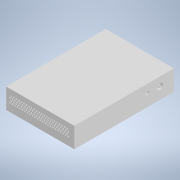
# Autodesk Inventor part: UBIQUITI EDGEROUTER-X
Saved by Autodesk Inventor 2020.2 (Build 242310000, 310)
## iProperties
Created: 2020-02-16
Part Number: UBIQUITI EDGEROUTER-X
Material: Generic
Document SubType Name: Modeling
Designer: mulve
Density: 1 g/cm^3
Appearance: Default
Author: mulve
Autodesk Inventor part; units mm, degrees
ref_plane "YZ Plane" through (0, 0, 0) normal (1, 0, 0) x (0, 1, 0)
ref_plane "XZ Plane" through (0, 0, 0) normal (0, 1, 0) x (-1, 0, 0)
sketch "Sketch1" plane through (0, 0, 0) normal (0, 1, 0) x (-1, 0, 0)
  line L0 (0, 0) -> (75.65, 0)
  line L1 (75.65, 0) -> (75.65, -110.31)
  line L2 (75.65, -110.31) -> (0, -110.31)
  line L3 (0, -110.31) -> (0, 0)
  dimension "d0" = 110.31
  dimension "d1" = 75.65
  constraints: 8 end point, 2 parallel, 1 horizontal, 1 perpendicular
  measures "d0" distance of L2.end L0.start
  measures "d1" distance of L1.end L2.end
extrude "Extrusion1" add sketch "Sketch1" along normal blind 22.5
sketch "Sketch2" plane through (0, 0, 0) normal (1, 0, 0) x (0, 0, -1)
  line L0 (0, 22.5) -> (110.31, 22.5) projected
  line L1 (0, 0) -> (0, 22.5) projected
  line L2 (110.31, 0) -> (110.31, 22.5) projected
  circle A0 centre (5.54, 15.27) radius 1.925
  circle A1 centre (104.77, 15.27) radius 1.925
  dimension "d4" = 7.23
  dimension "d5" = 7.23
  dimension "d6" = 5.54
  dimension "d7" = 5.54
  dimension "d8" = 3.85
  constraints: 2 centre point, 2 coincident, 1 equal radius
  measures "d4" distance from line of L0 point (5.54, 15.27)
  measures "d5" distance from line of L0 point (104.77, 15.27)
  measures "d6" distance from line of L1 point (5.54, 15.27)
  measures "d7" distance from line of L2 point (104.77, 15.27)
  measures "d8" diameter of A0
extrude "Extrusion2" cut sketch "Sketch2" against normal blind 0.1
sketch "Sketch3" plane through (0, 0, 0) normal (1, 0, 0) x (0, 0, -1)
  line L0 (0, 22.5) -> (110.31, 22.5) projected
  line L1 (0, 0) -> (0, 22.5) projected
  circle A0 centre (81.06, 13.3) radius 1.875
  dimension "d11" = 9.2
  dimension "d12" = 81.06
  dimension "d13" = 3.75
  constraints: 1 centre point, 1 coincident
  measures "d11" distance from line of L0 point (81.06, 13.3)
  measures "d12" distance from line of L1 point (81.06, 13.3)
  measures "d13" diameter of A0
extrude "Extrusion3" cut sketch "Sketch3" against normal blind 12.7
sketch "Sketch4" plane through (0, 0, 0) normal (1, 0, 0) x (0, 0, -1)
  line L0 (0, 0) -> (0, 22.5) projected
  line L1 (0, 22.5) -> (110.31, 22.5) projected
  circle A0 centre (13.8, 9.13) radius 1.5
  dimension "d16" = 13.8
  dimension "d17" = 13.37
  dimension "d18" = 3
  constraints: 1 centre point, 1 coincident
  measures "d16" distance from line of L0 point (13.8, 9.13)
  measures "d17" distance from line of L1 point (13.8, 9.13)
  measures "d18" diameter of A0
extrude "Extrusion4" cut sketch "Sketch4" against normal blind 0.2
sketch "Sketch5" plane through (0, 0, 0) normal (1, 0, 0) x (0, 0, -1)
  line L0 (90.8, 16.86) -> (99.47, 16.86)
  line L1 (99.47, 16.86) -> (99.47, 5.38)
  line L2 (99.47, 5.38) -> (90.8, 5.38)
  line L3 (90.8, 5.38) -> (90.8, 16.86)
  line L4 (110.31, 0) -> (110.31, 22.5) projected
  line L5 (0, 22.5) -> (110.31, 22.5) projected
  circle A0 centre (95.135, 12.62) radius 3.24
  circle A1 centre (95.135, 12.62) radius 1.125
  point P0 (0, 0)
  point P1 (95.135, 15.86)
  dimension "d25" = 6.48
  dimension "d21" = 8.67
  dimension "d22" = 10.84
  dimension "d23" = 11.48
  dimension "d24" = 5.64
  dimension "d26" = 1
  dimension "d27" = 2.25
  constraints: 8 end point, 2 coincident, 2 parallel, 1 centre point, 1 horizontal, 1 perpendicular, 1 vertical alignment, 2 other
  measures "d21" distance of L1.end L2.end
  measures "d22" distance between parallel lines of L4 L1
  measures "d23" distance of L0.end L1.end
  measures "d24" distance between parallel lines of L5 L0
  measures "d26" distance from line of L0 point (95.135, 15.86)
  measures "d27" diameter of A1
extrude "Extrusion5" cut sketch "Sketch5" against normal blind 9.2 contours A0
sketch "Sketch7" plane through (-75.65, 0, -110.31) normal (-1, 0, 0) x (0, 0, 1)
  line L0 (8.57, 5.39) -> (25.73, 5.39)
  line L1 (25.73, 5.39) -> (25.73, 19.5)
  line L2 (25.73, 19.5) -> (8.57, 19.5)
  line L3 (8.57, 19.5) -> (8.57, 5.39)
  line L4 (0, 22.5) -> (110.31, 22.5) projected
  line L5 (0, 0) -> (0, 22.5) projected
  line L6 (44.78, 5.39) -> (44.78, 19.5)
  line L7 (44.78, 19.5) -> (27.62, 19.5)
  line L8 (27.62, 19.5) -> (27.62, 5.39)
  line L9 (27.62, 5.39) -> (44.78, 5.39)
  line L10 (63.83, 5.39) -> (63.83, 19.5)
  line L11 (63.83, 19.5) -> (46.67, 19.5)
  line L12 (46.67, 19.5) -> (46.67, 5.39)
  line L13 (46.67, 5.39) -> (63.83, 5.39)
  line L14 (82.88, 5.39) -> (82.88, 19.5)
  line L15 (82.88, 19.5) -> (65.72, 19.5)
  line L16 (65.72, 19.5) -> (65.72, 5.39)
  line L17 (65.72, 5.39) -> (82.88, 5.39)
  line L18 (101.93, 5.39) -> (101.93, 19.5)
  line L19 (101.93, 19.5) -> (84.77, 19.5)
  line L20 (84.77, 19.5) -> (84.77, 5.39)
  line L21 (84.77, 5.39) -> (101.93, 5.39)
  point P0 (110.31, 0)
  dimension "d30" = 17.16
  dimension "d31" = 14.11
  dimension "d32" = 3
  dimension "d33" = 8.57
  dimension "d36" = 19.05
  constraints: 40 end point, 2 horizontal, 2 parallel, 1 perpendicular, 32 other
  measures "d30" distance of L1.end L2.end
  measures "d31" distance of L0.end L1.end
  measures "d32" distance between parallel lines of L4 L2
  measures "d33" distance between parallel lines of L5 L3
  measures "d36" distance of L0.end L6.start
extrude "Extrusion6" cut sketch "Sketch7" against normal blind 0.1
sketch "Sketch8" plane through (-75.55, 0, -110.31) normal (-1, 0, 0) x (0, 0, 1)
  line L0 (11.1, 7.46) -> (23.2, 7.46)
  line L1 (23.2, 7.46) -> (23.2, 14.99)
  line L2 (23.2, 14.99) -> (11.1, 14.99)
  line L3 (11.1, 14.99) -> (11.1, 7.46)
  line L4 (8.57, 5.39) -> (8.57, 19.5) projected
  line L5 (25.73, 19.5) -> (25.73, 5.39) projected
  line L6 (25.73, 5.39) -> (8.57, 5.39) projected
  line L7 (13.815, 7.46) -> (20.485, 7.46)
  line L8 (20.485, 7.46) -> (20.485, 16.67)
  line L9 (20.485, 16.67) -> (13.815, 16.67)
  line L10 (13.815, 16.67) -> (13.815, 7.46)
  line L11 (15.055, 7.46) -> (19.245, 7.46)
  line L12 (19.245, 7.46) -> (19.245, 18.23)
  line L13 (19.245, 18.23) -> (15.055, 18.23)
  line L14 (15.055, 18.23) -> (15.055, 7.46)
  line L15 (34.155, 18.23) -> (34.155, 7.46)
  line L16 (30.2, 14.99) -> (30.2, 7.46)
  line L17 (32.915, 16.67) -> (32.915, 7.46)
  line L18 (38.345, 7.46) -> (38.345, 18.23)
  line L19 (39.585, 7.46) -> (39.585, 16.67)
  line L20 (42.3, 7.46) -> (42.3, 14.99)
  line L21 (38.345, 18.23) -> (34.155, 18.23)
  line L22 (39.585, 16.67) -> (32.915, 16.67)
  line L23 (42.3, 14.99) -> (30.2, 14.99)
  line L24 (34.155, 7.46) -> (38.345, 7.46)
  line L25 (30.2, 7.46) -> (42.3, 7.46)
  line L26 (53.255, 18.23) -> (53.255, 7.46)
  line L27 (49.3, 14.99) -> (49.3, 7.46)
  line L28 (52.015, 16.67) -> (52.015, 7.46)
  line L29 (57.445, 7.46) -> (57.445, 18.23)
  line L30 (58.685, 7.46) -> (58.685, 16.67)
  line L31 (61.4, 7.46) -> (61.4, 14.99)
  line L32 (57.445, 18.23) -> (53.255, 18.23)
  line L33 (58.685, 16.67) -> (52.015, 16.67)
  line L34 (61.4, 14.99) -> (49.3, 14.99)
  line L35 (53.255, 7.46) -> (57.445, 7.46)
  line L36 (49.3, 7.46) -> (61.4, 7.46)
  line L37 (72.355, 18.23) -> (72.355, 7.46)
  line L38 (68.4, 14.99) -> (68.4, 7.46)
  line L39 (71.115, 16.67) -> (71.115, 7.46)
  line L40 (76.545, 7.46) -> (76.545, 18.23)
  line L41 (77.785, 7.46) -> (77.785, 16.67)
  line L42 (80.5, 7.46) -> (80.5, 14.99)
  line L43 (76.545, 18.23) -> (72.355, 18.23)
  line L44 (77.785, 16.67) -> (71.115, 16.67)
  line L45 (80.5, 14.99) -> (68.4, 14.99)
  line L46 (72.355, 7.46) -> (76.545, 7.46)
  line L47 (68.4, 7.46) -> (80.5, 7.46)
  line L48 (91.455, 18.23) -> (91.455, 7.46)
  line L49 (87.5, 14.99) -> (87.5, 7.46)
  line L50 (90.215, 16.67) -> (90.215, 7.46)
  line L51 (95.645, 7.46) -> (95.645, 18.23)
  line L52 (96.885, 7.46) -> (96.885, 16.67)
  line L53 (99.6, 7.46) -> (99.6, 14.99)
  line L54 (95.645, 18.23) -> (91.455, 18.23)
  line L55 (96.885, 16.67) -> (90.215, 16.67)
  line L56 (99.6, 14.99) -> (87.5, 14.99)
  line L57 (91.455, 7.46) -> (95.645, 7.46)
  line L58 (87.5, 7.46) -> (99.6, 7.46)
  point P0 (110.31, 0)
  point P1 (91.455, 16.67)
  point P2 (90.215, 14.99)
  point P3 (91.455, 7.46)
  point P4 (96.885, 14.99)
  point P5 (95.645, 16.67)
  point P6 (77.785, 14.99)
  point P7 (76.545, 16.67)
  point P8 (72.355, 16.67)
  point P9 (71.115, 14.99)
  point P10 (72.355, 7.46)
  point P11 (53.255, 7.46)
  point P12 (58.685, 14.99)
  point P13 (57.445, 16.67)
  point P14 (53.255, 16.67)
  point P15 (52.015, 14.99)
  point P16 (39.585, 14.99)
  point P17 (38.345, 16.67)
  point P18 (34.155, 16.67)
  point P19 (32.915, 14.99)
  point P20 (34.155, 7.46)
  point P21 (15.055, 16.67)
  point P22 (13.815, 14.99)
  point P23 (20.485, 14.99)
  point P24 (19.245, 16.67)
  dimension "d43" = 12.1
  dimension "d45" = 2.53
  dimension "d46" = 2.53
  dimension "d47" = 2.07
  dimension "d48" = 6.67
  dimension "d50" = 2.715
  dimension "d51" = 2.715
  dimension "d52" = 4.19
  dimension "d53" = 12.84
  dimension "d54" = 11.28
  dimension "d55" = 9.6
  dimension "d56" = 1.24
  dimension "d57" = 1.24
  dimension "d60" = 19.1
  constraints: 112 end point, 6 parallel, 6 point on line, 4 horizontal, 3 perpendicular, 1 collinear, 91 other
  measures "d43" distance of L0.start L0.end
  measures "d45" distance between parallel lines of L4 L3
  measures "d46" distance between parallel lines of L5 L1
  measures "d47" distance between parallel lines of L6 L0
  measures "d48" distance of L8.end L9.end
  measures "d50" distance between parallel lines of L3 L10
  measures "d51" distance between parallel lines of L1 L8
  measures "d52" distance of L12.end L13.end
  measures "d53" distance between parallel lines of L6 L13
  measures "d54" distance between parallel lines of L6 L9
  measures "d55" distance between parallel lines of L6 L2
  measures "d56" distance between parallel lines of L10 L14
  measures "d57" distance between parallel lines of L8 L12
  measures "d60" distance of L13.end L15.start
extrude "Extrusion7" cut sketch "Sketch8" against normal blind 15.75
sketch "Sketch9" plane through (0, 22.5, 0) normal (0, 1, 0) x (1, 0, 0)
  line L0 (0, 0) -> (0, 110.31) projected
  line L1 (0, 110.31) -> (-75.65, 110.31) projected
  circle A0 centre (-5.6, 88.05) radius 0.83
  circle A1 centre (-5.6, 74.79) radius 0.83
  circle A2 centre (-5.6, 65.06) radius 0.83
  circle A3 centre (-5.6, 55) radius 0.83
  circle A4 centre (-5.6, 45.05) radius 0.83
  circle A5 centre (-5.6, 34.75) radius 0.83
  dimension "d67" = 5.6
  dimension "d68" = 5.6
  dimension "d69" = 5.6
  dimension "d70" = 5.6
  dimension "d71" = 5.6
  dimension "d72" = 22.26
  dimension "d73" = 35.52
  dimension "d74" = 45.25
  dimension "d75" = 55.31
  dimension "d76" = 65.26
  dimension "d77" = 5.6
  dimension "d78" = 75.56
  dimension "d79" = 1.66
  constraints: 6 centre point, 6 coincident, 5 equal radius
  measures "d67" distance from line of L0 point (-5.6, 88.05)
  measures "d68" distance from line of L0 point (-5.6, 74.79)
  measures "d69" distance from line of L0 point (-5.6, 65.06)
  measures "d70" distance from line of L0 point (-5.6, 55)
  measures "d71" distance from line of L0 point (-5.6, 45.05)
  measures "d72" distance from line of L1 point (-5.6, 88.05)
  measures "d73" distance from line of L1 point (-5.6, 74.79)
  measures "d74" distance from line of L1 point (-5.6, 65.06)
  measures "d75" distance from line of L1 point (-5.6, 55)
  measures "d76" distance from line of L1 point (-5.6, 45.05)
  measures "d77" distance from line of L0 point (-5.6, 34.75)
  measures "d78" distance from line of L1 point (-5.6, 34.75)
  measures "d79" diameter of A0
extrude "Extrusion8" cut sketch "Sketch9" against normal blind 0.1
sketch "Sketch10" plane through (0, 0, 0) normal (0, -1, 0) x (1, 0, 0)
  line L0 (0, 0) -> (0, -110.31) projected
  line L1 (-75.65, 0) -> (0, 0) projected
  circle A0 centre (-9.5, -13.8) radius 4.3
  circle A1 centre (-9.5, -95.08) radius 4.3
  circle A2 centre (-55.22, -13.8) radius 4.3
  circle A3 centre (-55.22, -95.08) radius 4.3
  dimension "d82" = 9.5
  dimension "d83" = 13.8
  dimension "d84" = 8.6
  dimension "d87" = 81.28
  dimension "d90" = 45.72
  constraints: 4 centre point, 1 coincident, 1 horizontal, 1 vertical, 6 other
  measures "d82" distance from line of L0 point (-9.5, -13.8)
  measures "d83" distance from line of L1 point (-9.5, -13.8)
  measures "d84" diameter of A0
  measures "d87" distance of A0.centre A1.centre
  measures "d90" distance of A0.centre A2.centre
extrude "Extrusion9" cut sketch "Sketch10" against normal blind 0.33
sketch "Sketch11" plane through (-9.5, 0.33, -13.8) normal (0, -1, 0) x (1, 0, 0)
  circle A0 centre (0, 0) radius 3.825
  line L0 (9.5, 13.8) -> (9.5, -96.51) projected
  line L1 (9.5, -26.4546) -> (9.5, -62.5532)
  line L2 (-14.9441, 13.8) -> (-34.0604, 13.8)
  circle A1 centre (0, -81.3) radius 3.825
  circle A2 centre (-45.7, 0) radius 3.825
  circle A3 centre (-45.7, -81.3) radius 3.825
  dimension "d95" = 7.65
  dimension "d98" = 81.3
  dimension "d101" = 45.7
  constraints: 4 centre point, 4 end point, 2 horizontal, 2 point on line, 1 vertical, 6 other
  measures "d95" diameter of A0
  measures "d98" distance of A0.centre A1.centre
  measures "d101" distance of A0.centre A2.centre
extrude "Extrusion10" add sketch "Sketch11" along normal blind 1.91
fillet "Fillet1" radius 3.82 4 edges at (-13.325, -1.58, -13.8) (-59.025, -1.58, -13.8) (-13.325, -1.58, -95.1) (-59.025, -1.58, -95.1)
sketch "Sketch12" plane through (0, 0, 0) normal (0, -1, 0) x (1, 0, 0)
  line L0 (-34.3649, -13.3738) -> (-34.3649, -29.4338) construction
  line L1 (-32.3449, -15.3938) -> (-32.3449, -27.4138)
  line L2 (-36.3849, -27.4138) -> (-36.3849, -15.3938)
  arc A0 (-32.3449, -15.3938) -> (-36.3849, -15.3938) centre (-34.3649, -15.3938) ccw
  arc A1 (-36.3849, -27.4138) -> (-32.3449, -27.4138) centre (-34.3649, -27.4138) ccw
  line L3 (-42.3899, -21.4038) -> (-26.3399, -21.4038) construction
  line L4 (-40.3699, -23.4238) -> (-28.3599, -23.4238)
  line L5 (-28.3599, -19.3838) -> (-40.3699, -19.3838)
  arc A2 (-40.3699, -19.3838) -> (-40.3699, -23.4238) centre (-40.3699, -21.4038) ccw
  arc A3 (-28.3599, -23.4238) -> (-28.3599, -19.3838) centre (-28.3599, -21.4038) ccw
  circle A4 centre (-34.3649, -21.4038) radius 4
  line L6 (0, 0) -> (0, -110.31) construction
  line L7 (0, -55.155) -> (-75.6763, -55.155) construction
  line L8 (-75.55, -57.055) -> (-75.55, -52.865) construction
  line L9 (-34.3649, -96.9362) -> (-34.3649, -80.8762) construction
  line L10 (-32.3449, -94.9162) -> (-32.3449, -82.8962)
  line L11 (-36.3849, -82.8962) -> (-36.3849, -94.9162)
  arc A5 (-36.3849, -94.9162) -> (-32.3449, -94.9162) centre (-34.3649, -94.9162) ccw
  arc A6 (-32.3449, -82.8962) -> (-36.3849, -82.8962) centre (-34.3649, -82.8962) ccw
  line L12 (-42.3899, -88.9062) -> (-26.3399, -88.9062) construction
  line L13 (-40.3699, -86.8862) -> (-28.3599, -86.8862)
  line L14 (-28.3599, -90.9262) -> (-40.3699, -90.9262)
  arc A7 (-40.3699, -86.8862) -> (-40.3699, -90.9262) centre (-40.3699, -88.9062) ccw
  arc A8 (-28.3599, -90.9262) -> (-28.3599, -86.8862) centre (-28.3599, -88.9062) ccw
  circle A9 centre (-34.3649, -88.9062) radius 4
  point P0 (-29.4304, -19.3838)
  point P1 (-36.3849, -26.4943)
  point P2 (-29.4304, -90.9262)
  point P3 (-36.3849, -83.8157)
  point P4 (-36.3849, -85.4537)
  point P5 (-37.8174, -86.8862)
  point P6 (-37.8174, -90.9262)
  point P7 (-36.3849, -92.3586)
  point P8 (-32.3449, -92.3586)
  point P9 (-30.9124, -90.9262)
  point P10 (-30.9124, -86.8862)
  point P11 (-32.3449, -85.4537)
  point P12 (-30.9124, -19.3838)
  point P13 (-32.3449, -17.9514)
  point P14 (-36.3849, -17.9514)
  point P15 (-37.8174, -19.3838)
  point P16 (-37.8174, -23.4238)
  point P17 (-36.3849, -24.8563)
  point P18 (-32.3449, -24.8563)
  point P19 (-30.9124, -23.4238)
  dimension "d107" = 16.06
  dimension "d108" = 2.02
  dimension "d109" = 16.05
  dimension "d110" = 2.02
  dimension "d111" = 8.03
  dimension "d112" = 8
  dimension "d113" = 8.025
  constraints: 34 end point, 24 point on circle, 21 symmetric about line, 10 centre point, 8 point on line, 8 tangent, 3 midpoint, 2 coincident, 2 parallel, 2 perpendicular, 1 vertical, 5 other
  measures "d107" distance of L0.end L0.start
  measures "d108" horizontal distance of L0.end point (-36.385, -26.494)
  measures "d109" distance of L3.start L3.end
  measures "d110" vertical distance of L3.end point (-29.43, -19.384)
  measures "d111" vertical distance of L0.start L3.end
  measures "d112" diameter of A4
  measures "d113" horizontal distance of L0.start L3.end
extrude "Extrusion11" cut sketch "Sketch12" against normal blind 3.08
sketch "Sketch13" plane through (0, 3.08, 0) normal (0, -1, 0) x (1, 0, 0)
  line L0 (-23.1034, -9.3195) -> (-45.2023, -9.3195)
  line L1 (-45.2023, -9.3195) -> (-45.2023, -32.5345)
  line L2 (-45.2023, -32.5345) -> (-23.1034, -32.5345)
  line L3 (-23.1034, -32.5345) -> (-23.1034, -9.3195)
  line L4 (-23.1034, -102.1795) -> (-45.2023, -102.1795)
  line L5 (-45.2023, -102.1795) -> (-45.2023, -76.0626)
  line L6 (-45.2023, -76.0626) -> (-23.1034, -76.0626)
  line L7 (-23.1034, -76.0626) -> (-23.1034, -102.1795)
  point P0 (0, 0)
  constraints: 16 end point, 4 parallel, 2 horizontal, 2 perpendicular, 2 point on line
extrude "Extrusion12" cut sketch "Sketch13" along normal blind 2
sketch "Sketch14" plane through (-75.65, 0, 0) normal (0, 0, 1) x (1, 0, 0)
  line L0 (0, 22.5) -> (75.65, 22.5) projected
  line L1 (75.65, 0) -> (75.65, 22.5) projected
  circle A0 centre (67.58, 16.07) radius 0.8202
  circle A1 centre (64.76, 16.07) radius 0.8202
  circle A2 centre (61.94, 16.07) radius 0.8202
  circle A3 centre (59.12, 16.07) radius 0.8202
  circle A4 centre (56.3, 16.07) radius 0.8202
  circle A5 centre (53.48, 16.07) radius 0.8202
  circle A6 centre (50.66, 16.07) radius 0.8202
  circle A7 centre (47.84, 16.07) radius 0.8202
  circle A8 centre (45.02, 16.07) radius 0.8202
  circle A9 centre (42.2, 16.07) radius 0.8202
  circle A10 centre (39.38, 16.07) radius 0.8202
  circle A11 centre (36.56, 16.07) radius 0.8202
  circle A12 centre (33.74, 16.07) radius 0.8202
  circle A13 centre (30.92, 16.07) radius 0.8202
  circle A14 centre (28.1, 16.07) radius 0.8202
  circle A15 centre (25.28, 16.07) radius 0.8202
  circle A16 centre (22.46, 16.07) radius 0.8202
  circle A17 centre (19.64, 16.07) radius 0.8202
  circle A18 centre (16.82, 16.07) radius 0.8202
  circle A19 centre (14, 16.07) radius 0.8202
  circle A20 centre (11.18, 16.07) radius 0.8202
  circle A21 centre (8.36, 16.07) radius 0.8202
  circle A22 centre (5.54, 16.07) radius 0.8202
  circle A23 centre (67.58, 11.365) radius 0.8202
  circle A24 centre (64.76, 11.365) radius 0.8202
  circle A25 centre (61.94, 11.365) radius 0.8202
  circle A26 centre (59.12, 11.365) radius 0.8202
  circle A27 centre (56.3, 11.365) radius 0.8202
  circle A28 centre (53.48, 11.365) radius 0.8202
  circle A29 centre (50.66, 11.365) radius 0.8202
  circle A30 centre (47.84, 11.365) radius 0.8202
  circle A31 centre (45.02, 11.365) radius 0.8202
  circle A32 centre (42.2, 11.365) radius 0.8202
  circle A33 centre (39.38, 11.365) radius 0.8202
  circle A34 centre (36.56, 11.365) radius 0.8202
  circle A35 centre (33.74, 11.365) radius 0.8202
  circle A36 centre (30.92, 11.365) radius 0.8202
  circle A37 centre (28.1, 11.365) radius 0.8202
  circle A38 centre (25.28, 11.365) radius 0.8202
  circle A39 centre (22.46, 11.365) radius 0.8202
  circle A40 centre (19.64, 11.365) radius 0.8202
  circle A41 centre (16.82, 11.365) radius 0.8202
  circle A42 centre (14, 11.365) radius 0.8202
  circle A43 centre (11.18, 11.365) radius 0.8202
  circle A44 centre (8.36, 11.365) radius 0.8202
  circle A45 centre (5.54, 11.365) radius 0.8202
  circle A46 centre (68.85, 13.77) radius 0.8202
  circle A47 centre (66.03, 13.77) radius 0.8202
  circle A48 centre (63.21, 13.77) radius 0.8202
  circle A49 centre (60.39, 13.77) radius 0.8202
  circle A50 centre (57.57, 13.77) radius 0.8202
  circle A51 centre (54.75, 13.77) radius 0.8202
  circle A52 centre (51.93, 13.77) radius 0.8202
  circle A53 centre (49.11, 13.77) radius 0.8202
  circle A54 centre (46.29, 13.77) radius 0.8202
  circle A55 centre (43.47, 13.77) radius 0.8202
  circle A56 centre (40.65, 13.77) radius 0.8202
  circle A57 centre (37.83, 13.77) radius 0.8202
  circle A58 centre (35.01, 13.77) radius 0.8202
  circle A59 centre (32.19, 13.77) radius 0.8202
  circle A60 centre (29.37, 13.77) radius 0.8202
  circle A61 centre (26.55, 13.77) radius 0.8202
  circle A62 centre (23.73, 13.77) radius 0.8202
  circle A63 centre (20.91, 13.77) radius 0.8202
  circle A64 centre (18.09, 13.77) radius 0.8202
  circle A65 centre (15.27, 13.77) radius 0.8202
  circle A66 centre (12.45, 13.77) radius 0.8202
  circle A67 centre (9.63, 13.77) radius 0.8202
  circle A68 centre (6.81, 13.77) radius 0.8202
  circle A69 centre (3.99, 13.77) radius 0.8202
  circle A70 centre (68.85, 9.065) radius 0.8202
  circle A71 centre (66.03, 9.065) radius 0.8202
  circle A72 centre (63.21, 9.065) radius 0.8202
  circle A73 centre (60.39, 9.065) radius 0.8202
  circle A74 centre (57.57, 9.065) radius 0.8202
  circle A75 centre (54.75, 9.065) radius 0.8202
  circle A76 centre (51.93, 9.065) radius 0.8202
  circle A77 centre (49.11, 9.065) radius 0.8202
  circle A78 centre (46.29, 9.065) radius 0.8202
  circle A79 centre (43.47, 9.065) radius 0.8202
  circle A80 centre (40.65, 9.065) radius 0.8202
  circle A81 centre (37.83, 9.065) radius 0.8202
  circle A82 centre (35.01, 9.065) radius 0.8202
  circle A83 centre (32.19, 9.065) radius 0.8202
  circle A84 centre (29.37, 9.065) radius 0.8202
  circle A85 centre (26.55, 9.065) radius 0.8202
  circle A86 centre (23.73, 9.065) radius 0.8202
  circle A87 centre (20.91, 9.065) radius 0.8202
  circle A88 centre (18.09, 9.065) radius 0.8202
  circle A89 centre (15.27, 9.065) radius 0.8202
  circle A90 centre (12.45, 9.065) radius 0.8202
  circle A91 centre (9.63, 9.065) radius 0.8202
  circle A92 centre (6.81, 9.065) radius 0.8202
  circle A93 centre (3.99, 9.065) radius 0.8202
  point P0 (68.16, 16.65)
  point P1 (65.34, 16.65)
  point P2 (62.52, 16.65)
  point P3 (59.7, 16.65)
  point P4 (56.88, 16.65)
  point P5 (54.06, 16.65)
  point P6 (51.24, 16.65)
  point P7 (48.42, 16.65)
  point P8 (45.6, 16.65)
  point P9 (42.78, 16.65)
  point P10 (39.96, 16.65)
  point P11 (37.14, 16.65)
  point P12 (34.32, 16.65)
  point P13 (31.5, 16.65)
  point P14 (28.68, 16.65)
  point P15 (25.86, 16.65)
  point P16 (23.04, 16.65)
  point P17 (20.22, 16.65)
  point P18 (17.4, 16.65)
  point P19 (14.58, 16.65)
  point P20 (11.76, 16.65)
  point P21 (8.94, 16.65)
  point P22 (6.12, 16.65)
  point P23 (68.16, 11.945)
  point P24 (65.34, 11.945)
  point P25 (62.52, 11.945)
  point P26 (59.7, 11.945)
  point P27 (56.88, 11.945)
  point P28 (54.06, 11.945)
  point P29 (51.24, 11.945)
  point P30 (48.42, 11.945)
  point P31 (45.6, 11.945)
  point P32 (42.78, 11.945)
  point P33 (39.96, 11.945)
  point P34 (37.14, 11.945)
  point P35 (34.32, 11.945)
  point P36 (31.5, 11.945)
  point P37 (28.68, 11.945)
  point P38 (25.86, 11.945)
  point P39 (23.04, 11.945)
  point P40 (20.22, 11.945)
  point P41 (17.4, 11.945)
  point P42 (14.58, 11.945)
  point P43 (11.76, 11.945)
  point P44 (8.94, 11.945)
  point P45 (6.12, 11.945)
  point P46 (69.43, 14.35)
  point P47 (66.61, 14.35)
  point P48 (63.79, 14.35)
  point P49 (60.97, 14.35)
  point P50 (58.15, 14.35)
  point P51 (55.33, 14.35)
  point P52 (52.51, 14.35)
  point P53 (49.69, 14.35)
  point P54 (46.87, 14.35)
  point P55 (44.05, 14.35)
  point P56 (41.23, 14.35)
  point P57 (38.41, 14.35)
  point P58 (35.59, 14.35)
  point P59 (32.77, 14.35)
  point P60 (29.95, 14.35)
  point P61 (27.13, 14.35)
  point P62 (24.31, 14.35)
  point P63 (21.49, 14.35)
  point P64 (18.67, 14.35)
  point P65 (15.85, 14.35)
  point P66 (13.03, 14.35)
  point P67 (10.21, 14.35)
  point P68 (7.39, 14.35)
  point P69 (4.57, 14.35)
  point P70 (69.43, 9.645)
  point P71 (66.61, 9.645)
  point P72 (63.79, 9.645)
  point P73 (60.97, 9.645)
  point P74 (58.15, 9.645)
  point P75 (55.33, 9.645)
  point P76 (52.51, 9.645)
  point P77 (49.69, 9.645)
  point P78 (46.87, 9.645)
  point P79 (44.05, 9.645)
  point P80 (41.23, 9.645)
  point P81 (38.41, 9.645)
  point P82 (35.59, 9.645)
  point P83 (32.77, 9.645)
  point P84 (29.95, 9.645)
  point P85 (27.13, 9.645)
  point P86 (24.31, 9.645)
  point P87 (21.49, 9.645)
  point P88 (18.67, 9.645)
  point P89 (15.85, 9.645)
  point P90 (13.03, 9.645)
  point P91 (10.21, 9.645)
  point P92 (7.39, 9.645)
  point P93 (4.57, 9.645)
  dimension "d119" = 5.85
  dimension "d121" = 7.49
  dimension "d122" = 0.58
  dimension "d123" = 0.58
  dimension "d126" = 2.82
  dimension "d129" = 4.705
  dimension "d132" = 6.22
  dimension "d133" = 8.15
  dimension "d134" = 0.58
  dimension "d135" = 0.58
  dimension "d138" = 2.82
  dimension "d141" = 4.705
  constraints: 49 vertical, 47 horizontal, 2 coincident, 466 other
  measures "d119" distance from line of L0 point (68.16, 16.65)
  measures "d121" distance from line of L1 point (68.16, 16.65)
  measures "d122" horizontal distance of point (68.16, 16.65) point (67.58, 16.07)
  measures "d123" horizontal distance of point (68.16, 16.65) point (67.58, 16.07)
  measures "d126" distance of point (67.58, 16.07) point (64.76, 16.07)
  measures "d129" distance of point (67.58, 16.07) point (67.58, 11.365)
  measures "d132" distance from line of L1 point (69.43, 14.35)
  measures "d133" distance from line of L0 point (69.43, 14.35)
  measures "d134" horizontal distance of point (68.85, 13.77) point (69.43, 14.35)
  measures "d135" horizontal distance of point (68.85, 13.77) point (69.43, 14.35)
  measures "d138" distance of point (68.85, 13.77) point (66.03, 13.77)
  measures "d141" distance of point (68.85, 13.77) point (68.85, 9.065)
extrude "Extrusion13" cut sketch "Sketch14" against normal through all contours A0 | A1 | A2 | A3 | A4 | A5 | A6 | A7 | A8 | A9 | A10 | A11 | A12 | A13 | A14 | A15 | A16 | A17 | A18 | A23 | A24 | A25 | A26 | A27 | A28 | A29 | A30 | A31 | A32 | A33 | A34 | A35 | A36 | A37 | A38 | A39 | A40 | A41 | A46 | A47 | A48 | A49 | A50 | A51 | A52 | A53 | A54 | A55 | A56 | A57 | A58 | A59 | A60 | A61 | A62 | A63 | A64 | A70 | A71 | A72 | A73 | A74 | A75 | A76 | A77 | A78 | A79 | A80 | A81 | A82 | A83 | A84 | A85 | A86 | A87 | A88
extrude "Extrusion14" cut sketch "Sketch14" against normal blind 10.16 contours A19 | A20 | A21 | A22 | A42 | A43 | A44 | A45 | A65 | A66 | A67 | A68 | A69 | A89 | A90 | A91 | A92 | A93
ref_plane "Work Plane1" through (-75.65, 0, -55.155) normal (0, 0, 1) x (1, 0, 0)
mirror "Mirror1" about plane through (-75.65, 0, -55.155) normal (0, 0, 1) of "Extrusion14"
equation "\"d45\" = d46"
equation "\"d50\" = d51"
equation "\"d56\" = d57"
equation "\"d68\" = d67"
equation "\"d69\" = d68"
equation "\"d70\" = d69"
equation "\"d71\" = d70"
equation "\"d77\" = d71"
equation "\"d110\" = d108"
equation "\"d111\" = 0.5 * d107"
equation "\"d113\" = 0.5 * d109"
equation "\"d123\" = d122"
equation "\"d134\" = d123"
equation "\"d135\" = d134"
equation "\"d138\" = d126"
equation "\"d141\" = d129"
body "Solid1"
